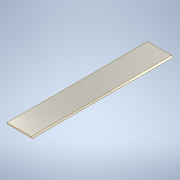
# Autodesk Inventor part: BLADE
Saved by Autodesk Inventor 2020 (Build 240168000, 168)
## iProperties
Created: 2019-11-06
Part Number: BLADE
Material: Titanium
Document SubType Name: Modeling
Designer: atmat
Density: 4.51 g/cm^3
Appearance: Titanium
Mass: 6350.08 g
Surface Area: 3741.3 cm^2
Volume: 1408 cm^3
Author: atmat
Autodesk Inventor part; units mm, degrees
ref_plane "YZ Plane" through (0, 0, 0) normal (1, 0, 0) x (0, 1, 0)
ref_plane "XZ Plane" through (0, 0, 0) normal (0, 1, 0) x (-1, 0, 0)
ref_plane "XY Plane" through (0, 0, 0) normal (0, 0, 1) x (1, 0, 0)
sketch "Sketch1" plane through (0, 0, 0) normal (0, 1, 0) x (-1, 0, 0)
  line L0 (9, 50) -> (-9, 50)
  line L1 (-9, 50) -> (-9, -50)
  line L2 (-9, -50) -> (9, -50)
  line L3 (9, -50) -> (9, 50)
  point P0 (0, 0)
  dimension "d0" = 18
  dimension "d1" = 9
  dimension "d2" = 100
  dimension "d3" = 50
  constraints: 8 end point, 2 parallel, 1 horizontal, 1 perpendicular
  measures "d0" distance of L0.start L0.end
  measures "d1" distance from line of L3 point (0, 0)
  measures "d2" distance of L2.end L0.start
  measures "d3" distance from line of point (0, 0) L0
extrude "Extrusion1" add sketch "Sketch1" along normal blind 0.8
chamfer "Chamfer1" distance 0.8 angle 45 1 edges at (9, 0.8, 0)
body "Solid1"
